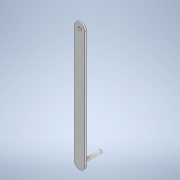
# Autodesk Inventor part: ramie cięgna traction loss
Saved by Autodesk Inventor 2021 (Build 250183000, 183)
## iProperties
Created: 2022-04-12
Part Number: ramie cięgna traction loss
Material: Generic
Document SubType Name: Modeling
Designer: Łukasz
Density: 1 g/cm^3
Appearance: Default
Author: Łukasz
Autodesk Inventor part; units mm, degrees
ref_plane "YZ Plane" through (0, 0, 0) normal (1, 0, 0) x (0, 1, 0)
ref_plane "XZ Plane" through (0, 0, 0) normal (0, 1, 0) x (-1, 0, 0)
ref_plane "XY Plane" through (0, 0, 0) normal (0, 0, 1) x (1, 0, 0)
sketch "Sketch1" plane through (0, 0, 0) normal (0, 0, 1) x (1, 0, 0)
  circle A0 centre (0, 0) radius 4
  circle A1 centre (0, 0) radius 12.5
  circle A2 centre (0, 280) radius 4
  circle A3 centre (0, 280) radius 12.5
  line L0 (12.5, 0) -> (12.5, 280)
  line L1 (-12.5, 280) -> (-12.5, 0)
  dimension "d0" = 8
  dimension "d1" = 25
  dimension "d2" = 280
  dimension "d3" = 0
  dimension "d4" = 8
  dimension "d5" = 25
  constraints: 4 centre point, 4 end point, 4 point on circle, 3 coincident, 3 tangent, 1 concentric, 1 vertical
  measures "d0" diameter of A0
  measures "d1" diameter of A1
  measures "d2" distance of point (0, 0) A2.centre
  measures "d3" horizontal distance of point (0, 0) A2.centre
  measures "d4" diameter of A2
  measures "d5" diameter of A3
extrude "Extrusion1" add sketch "Sketch1" along normal blind 4
sketch "Sketch2" plane through (0, 0, 4) normal (0, 0, 1) x (1, 0, 0)
  circle A0 centre (0, 0) radius 4 projected
extrude "Extrusion2" add sketch "Sketch2" against normal blind 50
equation "\"d4\" = d0"
equation "\"d5\" = d1"
body "Solid1"
